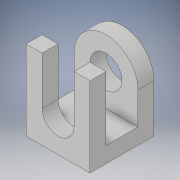
# Autodesk Inventor part: Part1
Saved by Autodesk Inventor 2018 (Build 220112000, 112)
## iProperties
Created: 2017-11-01
Part Number: Part1
Material: Generic
Document SubType Name: Modeling
Designer: kurtis
Density: 1 g/cm^3
Appearance: Default
Author: kurtis
Autodesk Inventor part; units mm, degrees
ref_plane "YZ Plane" through (0, 0, 0) normal (1, 0, 0) x (0, 1, 0)
ref_plane "XZ Plane" through (0, 0, 0) normal (0, 1, 0) x (-1, 0, 0)
ref_plane "XY Plane" through (0, 0, 0) normal (0, 0, 1) x (1, 0, 0)
sketch "Sketch1" plane through (0, 0, 0) normal (0, 0, 1) x (1, 0, 0)
  line L0 (0, 0) -> (20, 0)
  line L1 (20, 0) -> (20, 25)
  line L2 (20, 25) -> (15, 25)
  line L3 (15, 25) -> (15, 10)
  line L4 (10, 5) -> (10, 5)
  line L5 (5, 10) -> (5, 25)
  line L6 (5, 25) -> (0, 25)
  line L7 (0, 25) -> (0, 0)
  arc A0 (5, 10) -> (10, 5) centre (10, 10) ccw
  arc A1 (10, 5) -> (15, 10) centre (10, 10) ccw
  point P0 (15, 5)
  point P1 (5, 5)
  dimension "d0" = 20
  dimension "d1" = 25
  dimension "d2" = 5
  dimension "d3" = 20
  dimension "d4" = 10
  dimension "d5" = 5
  constraints: 16 end point, 6 perpendicular, 6 point on line, 4 point on circle, 4 tangent, 2 centre point, 1 concentric, 1 horizontal
  measures "d0" distance of L0.start L0.end
  measures "d1" distance of L0.end L1.end
  measures "d2" distance of L1.end L2.end
  measures "d3" distance of L2.end point (15, 5)
  measures "d4" distance of point (15, 5) point (5, 5)
  measures "d5" radius of A0
extrude "Extrusion1" add sketch "Sketch1" against normal blind 5
sketch "Sketch2" plane through (0, 0, -5) normal (0, 0, -1) x (-1, 0, 0)
  line L0 (0, 25) -> (0, 0) projected
  line L1 (-20, 25) -> (-20, 0) projected
  line L2 (0, 0) -> (-20, 0)
  line L3 (-20, 0) -> (-20, 5)
  line L4 (-20, 5) -> (0, 5)
  line L5 (0, 5) -> (0, 0)
  dimension "d8" = 5
  constraints: 8 end point, 2 parallel, 1 horizontal, 1 perpendicular, 1 point on line
  measures "d8" distance of L2.end L3.end
extrude "Extrusion2" add sketch "Sketch2" along normal blind 15
sketch "Sketch3" plane through (0, 0, -20) normal (0, 0, -1) x (-1, 0, 0)
  line L0 (-20, 25) -> (-20, 5) projected
  line L1 (0, 0) -> (-20, 0)
  line L2 (-20, 0) -> (-20, 15)
  line L3 (-10, 25) -> (-10, 25)
  line L4 (0, 15) -> (0, 0)
  arc A0 (-10, 25) -> (-20, 15) centre (-10, 15) ccw
  arc A1 (0, 15) -> (-10, 25) centre (-10, 15) ccw
  circle A2 centre (-10, 15) radius 5
  dimension "d11" = 10
  dimension "d12" = 10
  constraints: 8 end point, 4 point on circle, 4 tangent, 3 centre point, 2 parallel, 2 point on line, 1 coincident, 1 concentric, 1 horizontal, 1 perpendicular
  measures "d11" radius of A0
  measures "d12" diameter of A2
extrude "Extrusion3" add sketch "Sketch3" against normal blind 5
body "Solid1"
